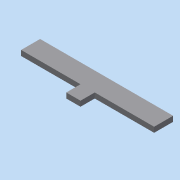
# Autodesk Inventor part: anillo3
Saved by Autodesk Inventor 2015 (Build 190159000, 159)
## iProperties
Created: 2017-09-29
Part Number: anillo3
Material: Generic
Document SubType Name: Modeling
Designer: macbook
Density: 1 g/cm^3
Appearance: Default
Author: macbook
Autodesk Inventor part; units mm, degrees
ref_plane "YZ Plane" through (0, 0, 0) normal (1, 0, 0) x (0, 1, 0)
ref_plane "XZ Plane" through (0, 0, 0) normal (0, 1, 0) x (-1, 0, 0)
ref_plane "XY Plane" through (0, 0, 0) normal (0, 0, 1) x (1, 0, 0)
sketch "Sketch1" plane through (0, 0, 0) normal (0, 0, 1) x (1, 0, 0)
  line L0 (0, 0) -> (100, 0)
  line L1 (-20, -20) -> (120, -20)
  line L2 (49.5, -20) -> (59.5, -20)
  line L3 (45, -20) -> (60, -20)
  line L4 (42.5, -20) -> (57.5, -20)
  line L5 (57.5, -20) -> (57.5, -35)
  line L6 (57.5, -35) -> (42.5, -35)
  line L7 (42.5, -35) -> (42.5, -20)
  line L8 (0, 0) -> (-20, 0)
  line L9 (-20, 0) -> (-20, -20)
  line L10 (100, 0) -> (120, 0)
  line L11 (120, 0) -> (120, -20)
  dimension "d0" = 15
  dimension "d1" = 15
  constraints: 24 end point, 6 horizontal, 4 point on line, 3 perpendicular, 2 parallel
  measures "d0" distance of L5.end L6.end
  measures "d1" distance of L5.start L5.end
extrude "Extrusion1" add sketch "Sketch1" along normal blind 5.5
body "Solid1"
